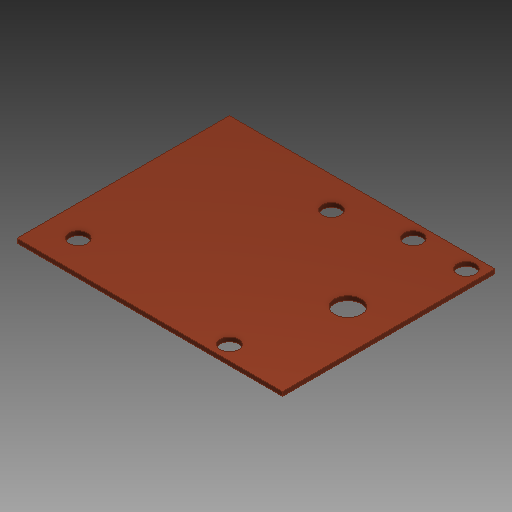
# Autodesk Inventor part: CU5
Saved by Autodesk Inventor 2019 (Build 230136000, 136)
## iProperties
Created: 2018-05-02
Part Number: CU5
Material: Copper
Document SubType Name: Modeling
Designer: Phil Erle
Density: 8.94 g/cm^3
Appearance: Copper - Satin
Author: Phil Erle
Autodesk Inventor part; units mm, degrees
ref_plane "YZ Plane" through (0, 0, 0) normal (1, 0, 0) x (0, 1, 0)
ref_plane "XZ Plane" through (0, 0, 0) normal (0, 1, 0) x (-1, 0, 0)
ref_plane "XY Plane" through (0, 0, 0) normal (0, 0, 1) x (1, 0, 0)
sketch "Sketch1" plane through (0, 0, 0) normal (0, 0, 1) x (1, 0, 0)
  line L0 (-32.5, -26) -> (32.5, -26)
  line L1 (32.5, -26) -> (32.5, 26)
  line L2 (32.5, 26) -> (-32.5, 26)
  line L3 (-32.5, 26) -> (-32.5, -26)
  line L4 (-32.5, -26) -> (32.5, 26) construction
  line L5 (32.5, -26) -> (-32.5, 26) construction
  point P0 (0, 0)
  dimension "d0" = 65
  dimension "d1" = 52
  constraints: 12 end point, 2 midpoint, 2 parallel, 1 horizontal, 1 perpendicular
  measures "d0" distance of L1.end L2.end
  measures "d1" distance of L2.end L0.start
extrude "Extrusion1" add sketch "Sketch1" along normal blind 1
sketch "Sketch4" plane through (0, 0, 1) normal (0, 0, 1) x (1, 0, 0)
  line L0 (29, -22.5) -> (16, -22.5) construction
  line L1 (16, -22.5) -> (16, 22.5) construction
  line L2 (16, 22.5) -> (29, 22.5) construction
  line L3 (29, 22.5) -> (29, -22.5) construction
  line L4 (29, -22.5) -> (16, 22.5) construction
  line L5 (16, -22.5) -> (29, 22.5) construction
  line L6 (32.5, -26) -> (32.5, 26) projected
  point P0 (0, 0)
  point P1 (22.5, 0)
  point P2 (22.5, 0)
  dimension "d20" = 13
  dimension "d31" = 3.5
  dimension "d32" = 45
  constraints: 12 end point, 3 coincident, 3 midpoint, 2 parallel, 1 horizontal, 1 horizontal alignment, 1 perpendicular
  measures "d20" distance of L1.end L2.end
  measures "d31" horizontal distance of L6.end L2.end
  measures "d32" distance of L2.end L0.start
hole "Hole3" at (16, 22.5, 1) at (29, 22.5, 1) at (16, -22.5, 1) direction (0, 0, -1) diameter 4.5 depth 8 tip angle 118 clearance for "Countersunk Flat Head Screw DIN EN ISO 2009" size "M4" standard "DIN"
sketch "Sketch5" plane through (0, 0, 1) normal (0, 0, 1) x (1, 0, 0)
  circle A0 centre (16, 22.5) radius 2.25 projected
  circle A1 centre (16, -22.5) radius 2.25 projected
  point P0 (0, 0)
  point P1 (-25, -18.5)
  point P2 (0, 18.5)
  dimension "d33" = 4
  dimension "d34" = 4
  dimension "d35" = 41
  dimension "d36" = 16
  measures "d33" vertical distance of A0.centre point (0, 18.5)
  measures "d34" vertical distance of A1.centre point (-25, -18.5)
  measures "d35" horizontal distance of A1.centre point (-25, -18.5)
  measures "d36" horizontal distance of A0.centre point (0, 18.5)
hole "Hole4" at (-25, -18.5, 1) at (0, 18.5, 1) direction (0, 0, -1) diameter 4.5 depth 8 tip angle 118 clearance for "Countersunk Flat Head Screw DIN EN ISO 2009" size "M4" standard "DIN"
sketch "Sketch6" plane through (0, 0, 1) normal (0, 0, 1) x (1, 0, 0)
  line L0 (32.5, -26) -> (32.5, 26) projected
  point P0 (0, 0)
  point P1 (22.5, 0)
  dimension "d44" = 10
  constraints: 1 horizontal alignment
  measures "d44" distance from line of L0 point (22.5, 0)
hole "Hole5" at (22.5, 0, 1) direction (0, 0, -1) diameter 6.6 depth 8 tip angle 118 clearance for "Countersunk Flat Head Screw DIN EN ISO 2009" size "M6" standard "DIN"
body "Solid1"
